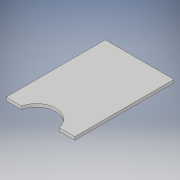
# Autodesk Inventor part: Plate 1
Saved by Autodesk Inventor 2019.4 (Build 234330000, 330)
## iProperties
Created: 2019-11-29
Part Number: Plate 1
Material: Generic
Document SubType Name: Modeling
Designer: admin
Density: 1 g/cm^3
Appearance: Default
Author: admin
Autodesk Inventor part; units mm, degrees
ref_plane "YZ Plane" through (0, 0, 0) normal (1, 0, 0) x (0, 1, 0)
ref_plane "XZ Plane" through (0, 0, 0) normal (0, 1, 0) x (-1, 0, 0)
ref_plane "XY Plane" through (0, 0, 0) normal (0, 0, 1) x (1, 0, 0)
sketch "Sketch1" plane through (0, 0, 0) normal (0, 1, 0) x (-1, 0, 0)
  line L0 (-45, 65) -> (45, 65)
  line L1 (45, 65) -> (45, -65)
  line L2 (45, -65) -> (-45, -65)
  line L3 (-45, -65) -> (-45, 65)
  line L4 (-45, 65) -> (45, -65) construction
  line L5 (45, 65) -> (-45, -65) construction
  point P0 (0, 0)
  dimension "d1" = 90
  dimension "d2" = 130
  constraints: 12 end point, 2 midpoint, 2 parallel, 1 horizontal, 1 perpendicular
  measures "d1" distance of L1.end L2.end
  measures "d2" distance of L0.end L1.end
extrude "Extrusion1" add sketch "Sketch1" along normal blind 4
sketch "Sketch2" plane through (0, 4, 0) normal (0, 1, 0) x (1, 0, 0)
  line L0 (-45, -65) -> (45, -65) projected
  arc A0 (24.4949, -65) -> (-24.4949, -65) centre (0, -70) ccw
  line L1 (0, -70) -> (0, 0) construction
  dimension "d5" = 25
  dimension "d6" = 5
  constraints: 2 end point, 2 point on circle, 2 point on line, 1 centre point, 1 coincident, 1 vertical
  measures "d5" radius of A0
  measures "d6" distance from line of L0 L1.start
extrude "Extrusion2" cut sketch "Sketch2" against normal blind 4
body "Solid1"
